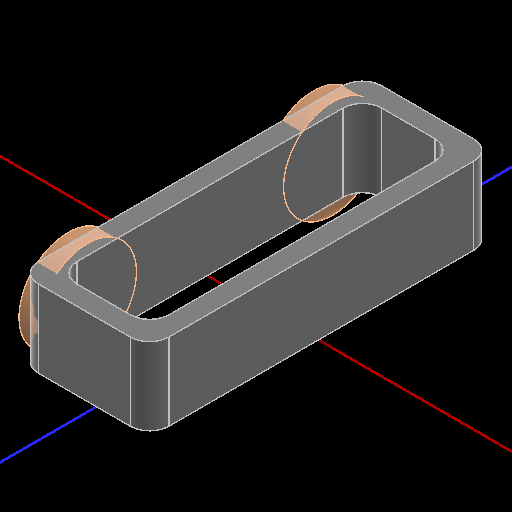
# Autodesk Inventor part: ziptie
Saved by Autodesk Inventor 2025.2 (Build 292293000, 293)
## iProperties
Created: 2025-11-17
Part Number: ziptie
Material: Acetal Resin, Black
Document SubType Name: Modeling
Designer: cloudy
Density: 1.425 g/cm^3
Appearance: Smooth - Black
Author: cloudy
Autodesk Inventor part; units mm, degrees
ref_plane "YZ Plane" through (0, 0, 0) normal (1, 0, 0) x (0, 1, 0)
ref_plane "XZ Plane" through (0, 0, 0) normal (0, 1, 0) x (-1, 0, 0)
ref_plane "XY Plane" through (0, 0, 0) normal (0, 0, 1) x (1, 0, 0)
sketch "Sketch1" plane through (0, 0, 0) normal (0, 1, 0) x (-1, 0, 0)
  line L0 (-3.3361, 9.3016) -> (3.4264, 9.3016)
  line L1 (3.4264, 9.3016) -> (3.4264, -8.4784)
  line L2 (3.4264, -8.4784) -> (-3.3361, -8.4784)
  line L3 (-3.3361, -8.4784) -> (-3.3361, 9.3016)
  line L4 (2.4264, -7.4784) -> (2.4264, 8.3016)
  line L5 (2.4264, 8.3016) -> (-2.3361, 8.3016)
  line L6 (-2.3361, 8.3016) -> (-2.3361, -7.4784)
  line L7 (-2.3361, -7.4784) -> (2.4264, -7.4784)
  point P0 (0, 0)
  dimension "d0" = 17.78
  dimension "d1" = 6.7625
  dimension "d2" = 1
  constraints: 16 end point, 4 parallel, 2 perpendicular, 1 horizontal, 3 other
  measures "d0" distance of L0.end L1.end
  measures "d1" distance of L1.end L2.end
  measures "d2" distance between parallel lines of L1 L4
extrude "Extrusion1" add sketch "Sketch1" along normal blind 4
fillet "Fillet1" radius 1 8 edges at (-3.4264, 2, 9.3016) (-3.4264, 2, -8.4784) (3.3361, 2, -8.4784) (3.3361, 2, 9.3016) (2.3361, 2, 8.3016) (-2.4264, 2, 8.3016) (-2.4264, 2, -7.4784) (2.3361, 2, -7.4784)
sketch "Sketch2" plane through (-2.4264, 0, -5.9384) normal (-1, 0, 0) x (0, 0, 1)
  circle A0 centre (0, 2) radius 2.54
  circle A1 centre (12.7, 2) radius 2.54
  line L0 (-1.54, 4) -> (14.24, 4) projected
  line L1 (15.24, 0) -> (15.24, 4) projected
  line L2 (15.24, 2) -> (-2.54, 2) construction
  line L3 (-2.54, 0) -> (-2.54, 4) projected
  dimension "d6" = 5.08
  dimension "d7" = 12.7
  constraints: 2 centre point, 2 end point, 2 midpoint, 2 point on line, 1 equal radius, 1 tangent
  measures "d6" diameter of A0
  measures "d7" distance of A1.centre A0.centre
surface extrude "ExtrusionSrf1" sketch "Sketch2" along normal up to surface (1 mm away) shown yes curves A0
surface extrude "ExtrusionSrf2" sketch "Sketch2" along normal up to surface (1 mm away) shown yes curves A1
body "Solid1"
body "Srf1"
body "Srf2"
